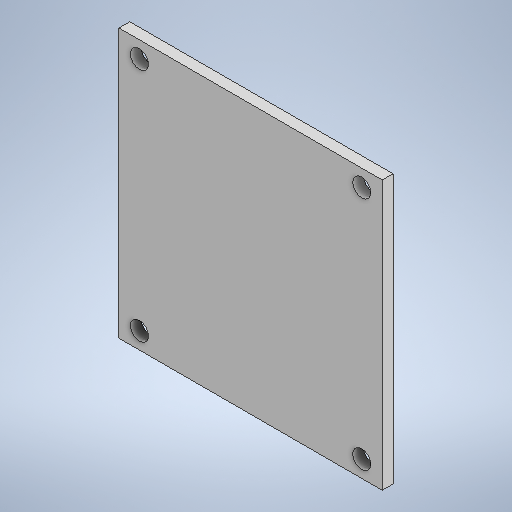
# Autodesk Inventor part: Pomodoro Robot Head's back
Saved by Autodesk Inventor 2025.3 (Build 293356030, 356C)
## iProperties
Created: 2026-07-18
Part Number: Pomodoro Robot Head's back
Material: Generic
Document SubType Name: Modeling
Designer: Samuel Correa Vega
Density: 1 g/cm^3
Appearance: Default
Author: Samuel Correa Vega
Autodesk Inventor part; units mm, degrees
ref_plane "YZ Plane" through (0, 0, 0) normal (1, 0, 0) x (0, 1, 0)
ref_plane "XZ Plane" through (0, 0, 0) normal (0, 1, 0) x (-1, 0, 0)
ref_plane "XY Plane" through (0, 0, 0) normal (0, 0, 1) x (1, 0, 0)
sketch "Sketch1" plane through (0, 0, 0) normal (0, 0, 1) x (1, 0, 0)
  line L0 (24.4, 24.9) -> (-24.4, 24.9)
  line L1 (-24.4, 24.9) -> (-24.4, -24.9)
  line L2 (-24.4, -24.9) -> (24.4, -24.9)
  line L3 (24.4, -24.9) -> (24.4, 24.9)
  circle A0 centre (20.6, 21.8) radius 1.675
  line L4 (0, 24.9) -> (0, -24.9) construction
  line L5 (24.4, 0) -> (-24.4, 0) construction
  circle A1 centre (-20.6, 21.8) radius 1.675
  line L6 (-24.4, 0) -> (24.4, 0) construction
  circle A2 centre (20.6, -21.8) radius 1.675
  circle A3 centre (-20.6, -21.8) radius 1.675
  point P0 (0, 0)
  dimension "d0" = 48.8
  dimension "d1" = 49.8
  dimension "d3" = 3.35
  dimension "d4" = 3.1
  dimension "d5" = 3.8
  constraints: 14 end point, 5 symmetric about line, 4 centre point, 4 midpoint, 2 parallel, 2 perpendicular, 1 horizontal, 1 horizontal alignment, 1 vertical alignment, 3 other
  measures "d0" distance of L0.start L0.end
  measures "d1" distance of L0.end L1.end
  measures "d3" diameter of A0
  measures "d4" distance from line of L0 A0.centre
  measures "d5" distance from line of L3 A0.centre
extrude "Extrusion1" add sketch "Sketch1" along normal blind 2
body "Solid1"
